Autodesk Inventor part; units mm, degrees
(part 3 of 4)
  arc A252 (17.6649, -16.827) -> (17.6214, -17.1875) centre (17.8848, -17.0365) ccw projected
  arc A253 (18.3289, -18.7127) -> (17.6214, -17.1875) centre (9.134, -22.0513) ccw projected
  arc A254 (17.8536, -19.1667) -> (18.3289, -18.7127) centre (0, 0) ccw projected
  arc A255 (16.3624, -18.39) -> (17.8536, -19.1667) centre (21.6099, -10.1343) ccw projected
  arc A256 (16.3624, -18.39) -> (16.0003, -18.4171) centre (16.1995, -18.6463) ccw projected
  arc A257 (15.9306, -18.4775) -> (16.0003, -18.4171) centre (0, 0) ccw projected
  arc A258 (15.9306, -18.4775) -> (15.8518, -18.8319) centre (16.1289, -18.7075) ccw projected
  arc A259 (16.4065, -20.4191) -> (15.8518, -18.8319) centre (6.9286, -22.8404) ccw projected
  arc A260 (15.889, -20.8243) -> (16.4065, -20.4191) centre (0, 0) ccw projected
  arc A261 (14.4811, -19.9053) -> (15.889, -20.8243) centre (20.5125, -12.2036) ccw projected
  arc A262 (14.4811, -19.9053) -> (14.1181, -19.8967) centre (14.2938, -20.1444) ccw projected
  arc A263 (14.0427, -19.95) -> (14.1181, -19.8967) centre (0, 0) ccw projected
  arc A264 (14.0427, -19.95) -> (13.9297, -20.295) centre (14.2175, -20.1983) ccw projected
  arc A265 (14.326, -21.9289) -> (13.9297, -20.295) centre (4.6565, -23.4096) ccw projected
  arc A266 (13.7713, -22.2814) -> (14.326, -21.9289) centre (0, 0) ccw projected
  arc A267 (12.4603, -21.2288) -> (13.7713, -22.2814) centre (19.2175, -14.1555) ccw projected
  arc A268 (12.4603, -21.2288) -> (12.0999, -21.1847) centre (12.2505, -21.4484) ccw projected
  arc A269 (12.0197, -21.2303) -> (12.0999, -21.1847) centre (0, 0) ccw projected
  arc A270 (12.0197, -21.2303) -> (11.8733, -21.5626) centre (12.1693, -21.4946) ccw projected
  arc A271 (12.1076, -23.2275) -> (11.8733, -21.5626) centre (2.3395, -23.7533) ccw projected
  arc A272 (11.5211, -23.524) -> (12.1076, -23.2275) centre (0, 0) ccw projected
  arc A273 (10.3195, -22.3479) -> (11.5211, -23.524) centre (17.7375, -15.9709) ccw projected
  arc A274 (10.3195, -22.3479) -> (9.9652, -22.2687) centre (10.0892, -22.5459) ccw projected
  arc A275 (9.8809, -22.3062) -> (9.9652, -22.2687) centre (0, 0) ccw projected
  arc A276 (9.8809, -22.3062) -> (9.7026, -22.6226) centre (10.0039, -22.5839) ccw projected
  arc A277 (9.7726, -24.3024) -> (9.7026, -22.6226) centre (0, -23.8682) ccw projected
  arc A278 (9.1598, -24.54) -> (9.7726, -24.3024) centre (0, 0) ccw projected
  arc A279 (8.0793, -23.2518) -> (9.1598, -24.54) centre (16.0867, -17.6326) ccw projected
  arc A280 (8.0793, -23.2518) -> (7.7345, -23.1382) centre (7.8307, -23.4262) ccw projected
  arc A281 (7.6469, -23.1673) -> (7.7345, -23.1382) centre (0, 0) ccw projected
  arc A282 (7.6469, -23.1673) -> (7.4385, -23.4646) centre (7.7421, -23.4557) ccw projected
  arc A283 (7.3435, -25.1433) -> (7.4385, -23.4646) centre (-2.3395, -23.7533) ccw projected
  arc A284 (6.7104, -25.3196) -> (7.3435, -25.1433) centre (0, 0) ccw projected
  arc A285 (5.7614, -23.9317) -> (6.7104, -25.3196) centre (14.2809, -19.1245) ccw projected
  arc A286 (5.7614, -23.9317) -> (5.4293, -23.7849) centre (5.4969, -24.081) ccw projected
  arc A287 (5.3393, -23.8053) -> (5.4293, -23.7849) centre (0, 0) ccw projected
  arc A288 (5.3393, -23.8053) -> (5.1028, -24.0808) centre (5.4057, -24.1016) ccw projected
  arc A289 (4.8437, -25.742) -> (5.1028, -24.0808) centre (-4.6565, -23.4096) ccw projected
  arc A290 (4.1963, -25.8554) -> (4.8437, -25.742) centre (0, 0) ccw projected
  arc A291 (3.3879, -24.3812) -> (4.1963, -25.8554) centre (12.3376, -20.4322) ccw projected
  arc A292 (3.3879, -24.3812) -> (3.0718, -24.2025) centre (3.11, -24.5038) ccw projected
  arc A293 (2.9802, -24.214) -> (3.0718, -24.2025) centre (0, 0) ccw projected
  arc A294 (2.9802, -24.214) -> (2.7179, -24.465) centre (3.0173, -24.5154) ccw projected
  arc A295 (2.2972, -26.0928) -> (2.7179, -24.465) centre (-6.9286, -22.8404) ccw projected
  arc A296 (1.6418, -26.1422) -> (2.2972, -26.0928) centre (0, 0) ccw projected
  arc A297 (0.9818, -24.5959) -> (1.6418, -26.1422) centre (10.2755, -21.5431) ccw projected
  arc A298 (0.9818, -24.5959) -> (0.6848, -24.3871) centre (0.6933, -24.6907) ccw projected
  arc A299 (0.5925, -24.3895) -> (0.6848, -24.3871) centre (0, 0) ccw projected
  arc A300 (0.5925, -24.3895) -> (0.3068, -24.6136) centre (0.5999, -24.6931) ccw projected
  arc A301 (-0.2714, -26.1923) -> (0.3068, -24.6136) centre (-9.134, -22.0513) ccw projected
  arc A302 (-0.9285, -26.1773) -> (-0.2714, -26.1923) centre (0, 0) ccw projected
  arc A303 (-1.4337, -24.5737) -> (-0.9285, -26.1773) centre (8.1145, -22.4465) ccw projected
  arc A304 (-1.4337, -24.5737) -> (-1.7089, -24.3368) centre (-1.7302, -24.6397) ccw projected
  arc A305 (-1.8009, -24.3301) -> (-1.7089, -24.3368) centre (0, 0) ccw projected
  arc A306 (-1.8009, -24.3301) -> (-2.1072, -24.5251) centre (-1.8234, -24.633) ccw projected
  arc A307 (-2.8374, -26.0396) -> (-2.1072, -24.5251) centre (-11.2514, -21.0499) ccw projected
  arc A308 (-3.4898, -25.9602) -> (-2.8374, -26.0396) centre (0, 0) ccw projected
  arc A309 (-3.8355, -24.3148) -> (-3.4898, -25.9602) centre (5.8752, -23.1338) ccw projected
  arc A310 (-3.8355, -24.3148) -> (-4.0861, -24.0521) centre (-4.137, -24.3515) ccw projected
  arc A311 (-4.177, -24.0365) -> (-4.0861, -24.0521) centre (0, 0) ccw projected
  arc A312 (-4.177, -24.0365) -> (-4.501, -24.2005) centre (-4.229, -24.3357) ccw projected
  arc A313 (-5.3761, -25.6361) -> (-4.501, -24.2005) centre (-13.2605, -19.8457) ccw projected
  arc A314 (-6.0176, -25.4932) -> (-5.3761, -25.6361) centre (0, 0) ccw projected
  arc A315 (-6.2003, -23.8218) -> (-6.0176, -25.4932) centre (3.5794, -23.5983) ccw projected
  arc A316 (-6.2003, -23.8218) -> (-6.4239, -23.5358) centre (-6.5039, -23.8287) ccw projected
  arc A317 (-6.5129, -23.5113) -> (-6.4239, -23.5358) centre (0, 0) ccw projected
  arc A318 (-6.5129, -23.5113) -> (-6.8514, -23.6428) centre (-6.594, -23.804) ccw projected
  arc A319 (-7.863, -24.9857) -> (-6.8514, -23.6428) centre (-15.1418, -18.4504) ccw projected
  arc A320 (-8.4873, -24.7806) -> (-7.863, -24.9857) centre (0, 0) ccw projected
  arc A321 (-8.5054, -23.0994) -> (-8.4873, -24.7806) centre (1.2492, -23.8355) ccw projected
  arc A322 (-8.5054, -23.0994) -> (-8.6999, -22.7928) centre (-8.8082, -23.0765) ccw projected
  arc A323 (-8.7861, -22.7597) -> (-8.6999, -22.7928) centre (0, 0) ccw projected
  arc A324 (-8.7861, -22.7597) -> (-9.1358, -22.8574) centre (-8.8954, -23.043) ccw projected
  arc A325 (-10.2741, -24.0947) -> (-9.1358, -22.8574) centre (-16.8774, -16.8774) ccw projected
  arc A326 (-10.8754, -23.8294) -> (-10.2741, -24.0947) centre (0, 0) ccw projected
  arc A327 (-10.7286, -22.1544) -> (-10.8754, -23.8294) centre (-1.0931, -23.8431) ccw projected
  arc A328 (-10.7286, -22.1544) -> (-10.8921, -21.8303) centre (-11.0277, -22.102) ccw projected
  arc A329 (-10.9746, -21.7889) -> (-10.8921, -21.8303) centre (0, 0) ccw projected
  arc A330 (-10.9746, -21.7889) -> (-11.3322, -21.8518) centre (-11.1112, -22.0602) ccw projected
  arc A331 (-12.5863, -22.9716) -> (-11.3322, -21.8518) centre (-18.4504, -15.1418) ccw projected
  arc A332 (-13.1587, -22.6486) -> (-12.5863, -22.9716) centre (0, 0) ccw projected
  arc A333 (-12.8484, -20.9962) -> (-13.1587, -22.6486) centre (-3.4249, -23.6212) ccw projected
  arc A334 (-12.8484, -20.9962) -> (-12.9794, -20.6576) centre (-13.141, -20.9147) ccw projected
  arc A335 (-13.0574, -20.6083) -> (-12.9794, -20.6576) centre (0, 0) ccw projected
  arc A336 (-13.0574, -20.6083) -> (-13.4195, -20.6359) centre (-13.22, -20.8648) ccw projected
  arc A337 (-14.7773, -21.6274) -> (-13.4195, -20.6359) centre (-19.8457, -13.2605) ccw projected
  arc A338 (-15.3153, -21.2498) -> (-14.7773, -21.6274) centre (0, 0) ccw projected
  arc A339 (-14.8445, -19.6357) -> (-15.3153, -21.2498) centre (-5.7237, -23.1717) ccw projected
  arc A340 (-14.8445, -19.6357) -> (-14.9417, -19.2859) centre (-15.1277, -19.5259) ccw projected
  arc A341 (-15.0145, -19.2292) -> (-14.9417, -19.2859) centre (0, 0) ccw projected
  arc A342 (-15.0145, -19.2292) -> (-15.3775, -19.2212) centre (-15.2014, -19.4686) ccw projected
  arc A343 (-16.826, -20.0748) -> (-15.3775, -19.2212) centre (-21.0499, -11.2514) ccw projected
  arc A344 (-17.3244, -19.6463) -> (-16.826, -20.0748) centre (0, 0) ccw projected
  arc A345 (-16.6977, -18.0862) -> (-17.3244, -19.6463) centre (-7.9674, -22.4991) ccw projected
  arc A346 (-16.6977, -18.0862) -> (-16.7601, -17.7285) centre (-16.9687, -17.9492) ccw projected
  arc A347 (-16.827, -17.6649) -> (-16.7601, -17.7285) centre (0, 0) ccw projected
  arc A348 (-16.827, -17.6649) -> (-17.1875, -17.6214) centre (-17.0365, -17.8848) ccw projected
  arc A349 (-18.7127, -18.3289) -> (-17.1875, -17.6214) centre (-22.0513, -9.134) ccw projected
  arc A350 (-19.1667, -17.8536) -> (-18.7127, -18.3289) centre (0, 0) ccw projected
  arc A351 (-18.39, -16.3624) -> (-19.1667, -17.8536) centre (-10.1343, -21.6099) ccw projected
  arc A352 (-18.39, -16.3624) -> (-18.4171, -16.0003) centre (-18.6463, -16.1995) ccw projected
  arc A353 (-18.4775, -15.9306) -> (-18.4171, -16.0003) centre (0, 0) ccw projected
  arc A354 (-18.4775, -15.9306) -> (-18.8319, -15.8518) centre (-18.7075, -16.1289) ccw projected
  arc A355 (-20.4191, -16.4065) -> (-18.8319, -15.8518) centre (-22.8404, -6.9286) ccw projected
  arc A356 (-20.8243, -15.889) -> (-20.4191, -16.4065) centre (0, 0) ccw projected
  arc A357 (-19.9053, -14.4811) -> (-20.8243, -15.889) centre (-12.2036, -20.5125) ccw projected
  arc A358 (-19.9053, -14.4811) -> (-19.8967, -14.1181) centre (-20.1444, -14.2938) ccw projected
  arc A359 (-19.95, -14.0427) -> (-19.8967, -14.1181) centre (0, 0) ccw projected
  arc A360 (-19.95, -14.0427) -> (-20.295, -13.9297) centre (-20.1983, -14.2175) ccw projected
  arc A361 (-21.9289, -14.326) -> (-20.295, -13.9297) centre (-23.4096, -4.6565) ccw projected
  arc A362 (-22.2814, -13.7713) -> (-21.9289, -14.326) centre (0, 0) ccw projected
  arc A363 (-21.2288, -12.4603) -> (-22.2814, -13.7713) centre (-14.1555, -19.2175) ccw projected
  arc A364 (-21.2288, -12.4603) -> (-21.1847, -12.0999) centre (-21.4484, -12.2505) ccw projected
  arc A365 (-21.2303, -12.0197) -> (-21.1847, -12.0999) centre (0, 0) ccw projected
  arc A366 (-21.2303, -12.0197) -> (-21.5626, -11.8733) centre (-21.4946, -12.1693) ccw projected
  arc A367 (-23.2275, -12.1076) -> (-21.5626, -11.8733) centre (-23.7533, -2.3395) ccw projected
  arc A368 (-23.524, -11.5211) -> (-23.2275, -12.1076) centre (0, 0) ccw projected
  arc A369 (-22.3479, -10.3195) -> (-23.524, -11.5211) centre (-15.9709, -17.7375) ccw projected
  arc A370 (-22.3479, -10.3195) -> (-22.2687, -9.9652) centre (-22.5459, -10.0892) ccw projected
  arc A371 (-22.3062, -9.8809) -> (-22.2687, -9.9652) centre (0, 0) ccw projected
  arc A372 (-22.3062, -9.8809) -> (-22.6226, -9.7026) centre (-22.5839, -10.0039) ccw projected
  arc A373 (-24.3024, -9.7726) -> (-22.6226, -9.7026) centre (-23.8682, 0) ccw projected
  arc A374 (-24.54, -9.1598) -> (-24.3024, -9.7726) centre (0, 0) ccw projected
  arc A375 (-23.2518, -8.0793) -> (-24.54, -9.1598) centre (-17.6326, -16.0867) ccw projected
  arc A376 (-23.2518, -8.0793) -> (-23.1382, -7.7345) centre (-23.4262, -7.8307) ccw projected
  arc A377 (-23.1673, -7.6469) -> (-23.1382, -7.7345) centre (0, 0) ccw projected
  arc A378 (-23.1673, -7.6469) -> (-23.4646, -7.4385) centre (-23.4557, -7.7421) ccw projected
  arc A379 (-25.1433, -7.3435) -> (-23.4646, -7.4385) centre (-23.7533, 2.3395) ccw projected
  arc A380 (-25.3196, -6.7104) -> (-25.1433, -7.3435) centre (0, 0) ccw projected
  arc A381 (-23.9317, -5.7614) -> (-25.3196, -6.7104) centre (-19.1245, -14.2809) ccw projected
  arc A382 (-23.9317, -5.7614) -> (-23.7849, -5.4293) centre (-24.081, -5.4969) ccw projected
  arc A383 (-23.8053, -5.3393) -> (-23.7849, -5.4293) centre (0, 0) ccw projected
  arc A384 (-23.8053, -5.3393) -> (-24.0808, -5.1028) centre (-24.1016, -5.4057) ccw projected
  point P0 (0, 0)
extrude "Extrusion5" add sketch "Sketch5" along normal blind 1.27
sketch "Sketch6" plane through (0, 0, 25.781) normal (0, 0, -1) x (-1, 0, 0)
  circle A0 centre (0, 0) radius 29.475
  constraints: 1 centre point, 1 coincident
extrude "Extrusion6" add sketch "Sketch6" along normal blind 1.27
sketch "Sketch7" plane through (0, 0, 32.131) normal (0, 0, 1) x (1, 0, 0)
  arc A0 (24.0808, -5.1028) -> (23.8053, -5.3393) centre (24.1016, -5.4057) ccw projected
  arc A1 (23.7849, -5.4293) -> (23.8053, -5.3393) centre (0, 0) ccw projected
  arc A2 (23.7849, -5.4293) -> (23.9317, -5.7614) centre (24.081, -5.4969) ccw projected
  arc A3 (25.3196, -6.7104) -> (23.9317, -5.7614) centre (19.1245, -14.2809) ccw projected
  arc A4 (25.1433, -7.3435) -> (25.3196, -6.7104) centre (0, 0) ccw projected
  arc A5 (23.4646, -7.4385) -> (25.1433, -7.3435) centre (23.7533, 2.3395) ccw projected
  arc A6 (23.4646, -7.4385) -> (23.1673, -7.6469) centre (23.4557, -7.7421) ccw projected
  arc A7 (23.1382, -7.7345) -> (23.1673, -7.6469) centre (0, 0) ccw projected
  arc A8 (23.1382, -7.7345) -> (23.2518, -8.0793) centre (23.4262, -7.8307) ccw projected
  arc A9 (24.54, -9.1598) -> (23.2518, -8.0793) centre (17.6326, -16.0867) ccw projected
  arc A10 (24.3024, -9.7726) -> (24.54, -9.1598) centre (0, 0) ccw projected
  arc A11 (22.6226, -9.7026) -> (24.3024, -9.7726) centre (23.8682, 0) ccw projected
  arc A12 (22.6226, -9.7026) -> (22.3062, -9.8809) centre (22.5839, -10.0039) ccw projected
  arc A13 (22.2687, -9.9652) -> (22.3062, -9.8809) centre (0, 0) ccw projected
  arc A14 (22.2687, -9.9652) -> (22.3479, -10.3195) centre (22.5459, -10.0892) ccw projected
  arc A15 (23.524, -11.5211) -> (22.3479, -10.3195) centre (15.9709, -17.7375) ccw projected
  arc A16 (23.2275, -12.1076) -> (23.524, -11.5211) centre (0, 0) ccw projected
  arc A17 (21.5626, -11.8733) -> (23.2275, -12.1076) centre (23.7533, -2.3395) ccw projected
  arc A18 (21.5626, -11.8733) -> (21.2303, -12.0197) centre (21.4946, -12.1693) ccw projected
  arc A19 (21.1847, -12.0999) -> (21.2303, -12.0197) centre (0, 0) ccw projected
  arc A20 (21.1847, -12.0999) -> (21.2288, -12.4603) centre (21.4484, -12.2505) ccw projected
  arc A21 (22.2814, -13.7713) -> (21.2288, -12.4603) centre (14.1555, -19.2175) ccw projected
  arc A22 (21.9289, -14.326) -> (22.2814, -13.7713) centre (0, 0) ccw projected
  arc A23 (20.295, -13.9297) -> (21.9289, -14.326) centre (23.4096, -4.6565) ccw projected
  arc A24 (20.295, -13.9297) -> (19.95, -14.0427) centre (20.1983, -14.2175) ccw projected
  arc A25 (19.8967, -14.1181) -> (19.95, -14.0427) centre (0, 0) ccw projected
  arc A26 (19.8967, -14.1181) -> (19.9053, -14.4811) centre (20.1444, -14.2938) ccw projected
  arc A27 (20.8243, -15.889) -> (19.9053, -14.4811) centre (12.2036, -20.5125) ccw projected
  arc A28 (20.4191, -16.4065) -> (20.8243, -15.889) centre (0, 0) ccw projected
  arc A29 (18.8319, -15.8518) -> (20.4191, -16.4065) centre (22.8404, -6.9286) ccw projected
  arc A30 (18.8319, -15.8518) -> (18.4775, -15.9306) centre (18.7075, -16.1289) ccw projected
  arc A31 (18.4171, -16.0003) -> (18.4775, -15.9306) centre (0, 0) ccw projected
  arc A32 (18.4171, -16.0003) -> (18.39, -16.3624) centre (18.6463, -16.1995) ccw projected
  arc A33 (19.1667, -17.8536) -> (18.39, -16.3624) centre (10.1343, -21.6099) ccw projected
  arc A34 (18.7127, -18.3289) -> (19.1667, -17.8536) centre (0, 0) ccw projected
  arc A35 (17.1875, -17.6214) -> (18.7127, -18.3289) centre (22.0513, -9.134) ccw projected
  arc A36 (17.1875, -17.6214) -> (16.827, -17.6649) centre (17.0365, -17.8848) ccw projected
  arc A37 (16.7601, -17.7285) -> (16.827, -17.6649) centre (0, 0) ccw projected
  arc A38 (16.7601, -17.7285) -> (16.6977, -18.0862) centre (16.9687, -17.9492) ccw projected
  arc A39 (17.3244, -19.6463) -> (16.6977, -18.0862) centre (7.9674, -22.4991) ccw projected
  arc A40 (16.826, -20.0748) -> (17.3244, -19.6463) centre (0, 0) ccw projected
  arc A41 (15.3775, -19.2212) -> (16.826, -20.0748) centre (21.0499, -11.2514) ccw projected
  arc A42 (15.3775, -19.2212) -> (15.0145, -19.2292) centre (15.2014, -19.4686) ccw projected
  arc A43 (14.9417, -19.2859) -> (15.0145, -19.2292) centre (0, 0) ccw projected
  arc A44 (14.9417, -19.2859) -> (14.8445, -19.6357) centre (15.1277, -19.5259) ccw projected
  arc A45 (15.3153, -21.2498) -> (14.8445, -19.6357) centre (5.7237, -23.1717) ccw projected
  arc A46 (14.7773, -21.6274) -> (15.3153, -21.2498) centre (0, 0) ccw projected
  arc A47 (13.4195, -20.6359) -> (14.7773, -21.6274) centre (19.8457, -13.2605) ccw projected
  arc A48 (13.4195, -20.6359) -> (13.0574, -20.6083) centre (13.22, -20.8648) ccw projected
  arc A49 (12.9794, -20.6576) -> (13.0574, -20.6083) centre (0, 0) ccw projected
  arc A50 (12.9794, -20.6576) -> (12.8484, -20.9962) centre (13.141, -20.9147) ccw projected
  arc A51 (13.1587, -22.6486) -> (12.8484, -20.9962) centre (3.4249, -23.6212) ccw projected
  arc A52 (12.5863, -22.9716) -> (13.1587, -22.6486) centre (0, 0) ccw projected
  arc A53 (11.3322, -21.8518) -> (12.5863, -22.9716) centre (18.4504, -15.1418) ccw projected
  arc A54 (11.3322, -21.8518) -> (10.9746, -21.7889) centre (11.1112, -22.0602) ccw projected
  arc A55 (10.8921, -21.8303) -> (10.9746, -21.7889) centre (0, 0) ccw projected
  arc A56 (10.8921, -21.8303) -> (10.7286, -22.1544) centre (11.0277, -22.102) ccw projected
  arc A57 (10.8754, -23.8294) -> (10.7286, -22.1544) centre (1.0931, -23.8431) ccw projected
  arc A58 (10.2741, -24.0947) -> (10.8754, -23.8294) centre (0, 0) ccw projected
  arc A59 (9.1358, -22.8574) -> (10.2741, -24.0947) centre (16.8774, -16.8774) ccw projected
  arc A60 (9.1358, -22.8574) -> (8.7861, -22.7597) centre (8.8954, -23.043) ccw projected
  arc A61 (8.6999, -22.7928) -> (8.7861, -22.7597) centre (0, 0) ccw projected
  arc A62 (8.6999, -22.7928) -> (8.5054, -23.0994) centre (8.8082, -23.0765) ccw projected
  arc A63 (8.4873, -24.7806) -> (8.5054, -23.0994) centre (-1.2492, -23.8355) ccw projected
  arc A64 (7.863, -24.9857) -> (8.4873, -24.7806) centre (0, 0) ccw projected
  arc A65 (6.8514, -23.6428) -> (7.863, -24.9857) centre (15.1418, -18.4504) ccw projected
  arc A66 (6.8514, -23.6428) -> (6.5129, -23.5113) centre (6.594, -23.804) ccw projected
  arc A67 (6.4239, -23.5358) -> (6.5129, -23.5113) centre (0, 0) ccw projected
  arc A68 (6.4239, -23.5358) -> (6.2003, -23.8218) centre (6.5039, -23.8287) ccw projected
  arc A69 (6.0176, -25.4932) -> (6.2003, -23.8218) centre (-3.5794, -23.5983) ccw projected
  arc A70 (5.3761, -25.6361) -> (6.0176, -25.4932) centre (0, 0) ccw projected
  arc A71 (4.501, -24.2005) -> (5.3761, -25.6361) centre (13.2605, -19.8457) ccw projected
  arc A72 (4.501, -24.2005) -> (4.177, -24.0365) centre (4.229, -24.3357) ccw projected
  arc A73 (4.0861, -24.0521) -> (4.177, -24.0365) centre (0, 0) ccw projected
  arc A74 (4.0861, -24.0521) -> (3.8355, -24.3148) centre (4.137, -24.3515) ccw projected
  arc A75 (3.4898, -25.9602) -> (3.8355, -24.3148) centre (-5.8752, -23.1338) ccw projected
  arc A76 (2.8374, -26.0396) -> (3.4898, -25.9602) centre (0, 0) ccw projected
  arc A77 (2.1072, -24.5251) -> (2.8374, -26.0396) centre (11.2514, -21.0499) ccw projected
  arc A78 (2.1072, -24.5251) -> (1.8009, -24.3301) centre (1.8234, -24.633) ccw projected
  arc A79 (1.7089, -24.3368) -> (1.8009, -24.3301) centre (0, 0) ccw projected
  arc A80 (1.7089, -24.3368) -> (1.4337, -24.5737) centre (1.7302, -24.6397) ccw projected
  arc A81 (0.9285, -26.1773) -> (1.4337, -24.5737) centre (-8.1145, -22.4465) ccw projected
  arc A82 (0.2714, -26.1923) -> (0.9285, -26.1773) centre (0, 0) ccw projected
  arc A83 (-0.3068, -24.6136) -> (0.2714, -26.1923) centre (9.134, -22.0513) ccw projected
  arc A84 (-0.3068, -24.6136) -> (-0.5925, -24.3895) centre (-0.5999, -24.6931) ccw projected
  arc A85 (-0.6848, -24.3871) -> (-0.5925, -24.3895) centre (0, 0) ccw projected
  arc A86 (-0.6848, -24.3871) -> (-0.9818, -24.5959) centre (-0.6933, -24.6907) ccw projected
  arc A87 (-1.6418, -26.1422) -> (-0.9818, -24.5959) centre (-10.2755, -21.5431) ccw projected
  arc A88 (-2.2972, -26.0928) -> (-1.6418, -26.1422) centre (0, 0) ccw projected
  arc A89 (-2.7179, -24.465) -> (-2.2972, -26.0928) centre (6.9286, -22.8404) ccw projected
  arc A90 (-2.7179, -24.465) -> (-2.9802, -24.214) centre (-3.0173, -24.5154) ccw projected
  arc A91 (-3.0718, -24.2025) -> (-2.9802, -24.214) centre (0, 0) ccw projected
  arc A92 (-3.0718, -24.2025) -> (-3.3879, -24.3812) centre (-3.11, -24.5038) ccw projected
  arc A93 (-4.1963, -25.8554) -> (-3.3879, -24.3812) centre (-12.3376, -20.4322) ccw projected
  arc A94 (-4.8437, -25.742) -> (-4.1963, -25.8554) centre (0, 0) ccw projected
  arc A95 (-5.1028, -24.0808) -> (-4.8437, -25.742) centre (4.6565, -23.4096) ccw projected
  arc A96 (-5.1028, -24.0808) -> (-5.3393, -23.8053) centre (-5.4057, -24.1016) ccw projected
  arc A97 (-5.4293, -23.7849) -> (-5.3393, -23.8053) centre (0, 0) ccw projected
  arc A98 (-5.4293, -23.7849) -> (-5.7614, -23.9317) centre (-5.4969, -24.081) ccw projected
  arc A99 (-6.7104, -25.3196) -> (-5.7614, -23.9317) centre (-14.2809, -19.1245) ccw projected
  arc A100 (-7.3435, -25.1433) -> (-6.7104, -25.3196) centre (0, 0) ccw projected
  arc A101 (-7.4385, -23.4646) -> (-7.3435, -25.1433) centre (2.3395, -23.7533) ccw projected
  arc A102 (-7.4385, -23.4646) -> (-7.6469, -23.1673) centre (-7.7421, -23.4557) ccw projected
  arc A103 (-7.7345, -23.1382) -> (-7.6469, -23.1673) centre (0, 0) ccw projected
  arc A104 (-7.7345, -23.1382) -> (-8.0793, -23.2518) centre (-7.8307, -23.4262) ccw projected
  arc A105 (-9.1598, -24.54) -> (-8.0793, -23.2518) centre (-16.0867, -17.6326) ccw projected
  arc A106 (-9.7726, -24.3024) -> (-9.1598, -24.54) centre (0, 0) ccw projected
  arc A107 (-9.7026, -22.6226) -> (-9.7726, -24.3024) centre (0, -23.8682) ccw projected
  arc A108 (-9.7026, -22.6226) -> (-9.8809, -22.3062) centre (-10.0039, -22.5839) ccw projected
  arc A109 (-9.9652, -22.2687) -> (-9.8809, -22.3062) centre (0, 0) ccw projected
  arc A110 (-9.9652, -22.2687) -> (-10.3195, -22.3479) centre (-10.0892, -22.5459) ccw projected
  arc A111 (-11.5211, -23.524) -> (-10.3195, -22.3479) centre (-17.7375, -15.9709) ccw projected
  arc A112 (-12.1076, -23.2275) -> (-11.5211, -23.524) centre (0, 0) ccw projected
  arc A113 (-11.8733, -21.5626) -> (-12.1076, -23.2275) centre (-2.3395, -23.7533) ccw projected
  arc A114 (-11.8733, -21.5626) -> (-12.0197, -21.2303) centre (-12.1693, -21.4946) ccw projected
  arc A115 (-12.0999, -21.1847) -> (-12.0197, -21.2303) centre (0, 0) ccw projected
  arc A116 (-12.0999, -21.1847) -> (-12.4603, -21.2288) centre (-12.2505, -21.4484) ccw projected
  arc A117 (-13.7713, -22.2814) -> (-12.4603, -21.2288) centre (-19.2175, -14.1555) ccw projected
  arc A118 (-14.326, -21.9289) -> (-13.7713, -22.2814) centre (0, 0) ccw projected
  arc A119 (-13.9297, -20.295) -> (-14.326, -21.9289) centre (-4.6565, -23.4096) ccw projected
  arc A120 (-13.9297, -20.295) -> (-14.0427, -19.95) centre (-14.2175, -20.1983) ccw projected
  arc A121 (-14.1181, -19.8967) -> (-14.0427, -19.95) centre (0, 0) ccw projected
  arc A122 (-14.1181, -19.8967) -> (-14.4811, -19.9053) centre (-14.2938, -20.1444) ccw projected
  arc A123 (-15.889, -20.8243) -> (-14.4811, -19.9053) centre (-20.5125, -12.2036) ccw projected
  arc A124 (-16.4065, -20.4191) -> (-15.889, -20.8243) centre (0, 0) ccw projected
  arc A125 (-15.8518, -18.8319) -> (-16.4065, -20.4191) centre (-6.9286, -22.8404) ccw projected
  arc A126 (-15.8518, -18.8319) -> (-15.9306, -18.4775) centre (-16.1289, -18.7075) ccw projected
  arc A127 (-16.0003, -18.4171) -> (-15.9306, -18.4775) centre (0, 0) ccw projected
  arc A128 (-16.0003, -18.4171) -> (-16.3624, -18.39) centre (-16.1995, -18.6463) ccw projected
  arc A129 (-17.8536, -19.1667) -> (-16.3624, -18.39) centre (-21.6099, -10.1343) ccw projected
  arc A130 (-18.3289, -18.7127) -> (-17.8536, -19.1667) centre (0, 0) ccw projected
  arc A131 (-17.6214, -17.1875) -> (-18.3289, -18.7127) centre (-9.134, -22.0513) ccw projected
  arc A132 (-17.6214, -17.1875) -> (-17.6649, -16.827) centre (-17.8848, -17.0365) ccw projected
  arc A133 (-17.7285, -16.7601) -> (-17.6649, -16.827) centre (0, 0) ccw projected
  arc A134 (-17.7285, -16.7601) -> (-18.0862, -16.6977) centre (-17.9492, -16.9687) ccw projected
  arc A135 (-19.6463, -17.3244) -> (-18.0862, -16.6977) centre (-22.4991, -7.9674) ccw projected
  arc A136 (-20.0748, -16.826) -> (-19.6463, -17.3244) centre (0, 0) ccw projected
  arc A137 (-19.2212, -15.3775) -> (-20.0748, -16.826) centre (-11.2514, -21.0499) ccw projected
  arc A138 (-19.2212, -15.3775) -> (-19.2292, -15.0145) centre (-19.4686, -15.2014) ccw projected
  arc A139 (-19.2859, -14.9417) -> (-19.2292, -15.0145) centre (0, 0) ccw projected
  arc A140 (-19.2859, -14.9417) -> (-19.6357, -14.8445) centre (-19.5259, -15.1277) ccw projected
  arc A141 (-21.2498, -15.3153) -> (-19.6357, -14.8445) centre (-23.1717, -5.7237) ccw projected
  arc A142 (-21.6274, -14.7773) -> (-21.2498, -15.3153) centre (0, 0) ccw projected
  arc A143 (-20.6359, -13.4195) -> (-21.6274, -14.7773) centre (-13.2605, -19.8457) ccw projected
  arc A144 (-20.6359, -13.4195) -> (-20.6083, -13.0574) centre (-20.8648, -13.22) ccw projected
  arc A145 (-20.6576, -12.9794) -> (-20.6083, -13.0574) centre (0, 0) ccw projected
  arc A146 (-20.6576, -12.9794) -> (-20.9962, -12.8484) centre (-20.9147, -13.141) ccw projected
  arc A147 (-22.6486, -13.1587) -> (-20.9962, -12.8484) centre (-23.6212, -3.4249) ccw projected
  arc A148 (-22.9716, -12.5863) -> (-22.6486, -13.1587) centre (0, 0) ccw projected
  arc A149 (-21.8518, -11.3322) -> (-22.9716, -12.5863) centre (-15.1418, -18.4504) ccw projected
  arc A150 (-21.8518, -11.3322) -> (-21.7889, -10.9746) centre (-22.0602, -11.1112) ccw projected
  arc A151 (-21.8303, -10.8921) -> (-21.7889, -10.9746) centre (0, 0) ccw projected
  arc A152 (-21.8303, -10.8921) -> (-22.1544, -10.7286) centre (-22.102, -11.0277) ccw projected
  arc A153 (-23.8294, -10.8754) -> (-22.1544, -10.7286) centre (-23.8431, -1.0931) ccw projected
  arc A154 (-24.0947, -10.2741) -> (-23.8294, -10.8754) centre (0, 0) ccw projected
  arc A155 (-22.8574, -9.1358) -> (-24.0947, -10.2741) centre (-16.8774, -16.8774) ccw projected
  arc A156 (-22.8574, -9.1358) -> (-22.7597, -8.7861) centre (-23.043, -8.8954) ccw projected
  arc A157 (-22.7928, -8.6999) -> (-22.7597, -8.7861) centre (0, 0) ccw projected
  arc A158 (-22.7928, -8.6999) -> (-23.0994, -8.5054) centre (-23.0765, -8.8082) ccw projected
  arc A159 (-24.7806, -8.4873) -> (-23.0994, -8.5054) centre (-23.8355, 1.2492) ccw projected
  arc A160 (-24.9857, -7.863) -> (-24.7806, -8.4873) centre (0, 0) ccw projected
  arc A161 (-23.6428, -6.8514) -> (-24.9857, -7.863) centre (-18.4504, -15.1418) ccw projected
  arc A162 (-23.6428, -6.8514) -> (-23.5113, -6.5129) centre (-23.804, -6.594) ccw projected
  arc A163 (-23.5358, -6.4239) -> (-23.5113, -6.5129) centre (0, 0) ccw projected
  arc A164 (-23.5358, -6.4239) -> (-23.8218, -6.2003) centre (-23.8287, -6.5039) ccw projected
  arc A165 (-25.4932, -6.0176) -> (-23.8218, -6.2003) centre (-23.5983, 3.5794) ccw projected
  arc A166 (-25.6361, -5.3761) -> (-25.4932, -6.0176) centre (0, 0) ccw projected
  arc A167 (-24.2005, -4.501) -> (-25.6361, -5.3761) centre (-19.8457, -13.2605) ccw projected
  arc A168 (-24.2005, -4.501) -> (-24.0365, -4.177) centre (-24.3357, -4.229) ccw projected
  arc A169 (-24.0521, -4.0861) -> (-24.0365, -4.177) centre (0, 0) ccw projected
  arc A170 (-24.0521, -4.0861) -> (-24.3148, -3.8355) centre (-24.3515, -4.137) ccw projected
  arc A171 (-25.9602, -3.4898) -> (-24.3148, -3.8355) centre (-23.1338, 5.8752) ccw projected
  arc A172 (-26.0396, -2.8374) -> (-25.9602, -3.4898) centre (0, 0) ccw projected
  arc A173 (-24.5251, -2.1072) -> (-26.0396, -2.8374) centre (-21.0499, -11.2514) ccw projected
  arc A174 (-24.5251, -2.1072) -> (-24.3301, -1.8009) centre (-24.633, -1.8234) ccw projected
  arc A175 (-24.3368, -1.7089) -> (-24.3301, -1.8009) centre (0, 0) ccw projected
  arc A176 (-24.3368, -1.7089) -> (-24.5737, -1.4337) centre (-24.6397, -1.7302) ccw projected
  arc A177 (-26.1773, -0.9285) -> (-24.5737, -1.4337) centre (-22.4465, 8.1145) ccw projected
  arc A178 (-26.1923, -0.2714) -> (-26.1773, -0.9285) centre (0, 0) ccw projected
  arc A179 (-24.6136, 0.3068) -> (-26.1923, -0.2714) centre (-22.0513, -9.134) ccw projected
  arc A180 (-24.6136, 0.3068) -> (-24.3895, 0.5925) centre (-24.6931, 0.5999) ccw projected
  arc A181 (-24.3871, 0.6848) -> (-24.3895, 0.5925) centre (0, 0) ccw projected
  arc A182 (-24.3871, 0.6848) -> (-24.5959, 0.9818) centre (-24.6907, 0.6933) ccw projected
  arc A183 (-26.1422, 1.6418) -> (-24.5959, 0.9818) centre (-21.5431, 10.2755) ccw projected
  arc A184 (-26.0928, 2.2972) -> (-26.1422, 1.6418) centre (0, 0) ccw projected
  arc A185 (-24.465, 2.7179) -> (-26.0928, 2.2972) centre (-22.8404, -6.9286) ccw projected
  arc A186 (-24.465, 2.7179) -> (-24.214, 2.9802) centre (-24.5154, 3.0173) ccw projected
  arc A187 (-24.2025, 3.0718) -> (-24.214, 2.9802) centre (0, 0) ccw projected
  arc A188 (-24.2025, 3.0718) -> (-24.3812, 3.3879) centre (-24.5038, 3.11) ccw projected
  arc A189 (-25.8554, 4.1963) -> (-24.3812, 3.3879) centre (-20.4322, 12.3376) ccw projected
  arc A190 (-25.742, 4.8437) -> (-25.8554, 4.1963) centre (0, 0) ccw projected
  arc A191 (-24.0808, 5.1028) -> (-25.742, 4.8437) centre (-23.4096, -4.6565) ccw projected
  arc A192 (-24.0808, 5.1028) -> (-23.8053, 5.3393) centre (-24.1016, 5.4057) ccw projected
  arc A193 (-23.7849, 5.4293) -> (-23.8053, 5.3393) centre (0, 0) ccw projected
  arc A194 (-23.7849, 5.4293) -> (-23.9317, 5.7614) centre (-24.081, 5.4969) ccw projected
  arc A195 (-25.3196, 6.7104) -> (-23.9317, 5.7614) centre (-19.1245, 14.2809) ccw projected
  arc A196 (-25.1433, 7.3435) -> (-25.3196, 6.7104) centre (0, 0) ccw projected
  arc A197 (-23.4646, 7.4385) -> (-25.1433, 7.3435) centre (-23.7533, -2.3395) ccw projected
  arc A198 (-23.4646, 7.4385) -> (-23.1673, 7.6469) centre (-23.4557, 7.7421) ccw projected
  arc A199 (-23.1382, 7.7345) -> (-23.1673, 7.6469) centre (0, 0) ccw projected
  arc A200 (-23.1382, 7.7345) -> (-23.2518, 8.0793) centre (-23.4262, 7.8307) ccw projected
  arc A201 (-24.54, 9.1598) -> (-23.2518, 8.0793) centre (-17.6326, 16.0867) ccw projected
  arc A202 (-24.3024, 9.7726) -> (-24.54, 9.1598) centre (0, 0) ccw projected
  arc A203 (-22.6226, 9.7026) -> (-24.3024, 9.7726) centre (-23.8682, 0) ccw projected
  arc A204 (-22.6226, 9.7026) -> (-22.3062, 9.8809) centre (-22.5839, 10.0039) ccw projected
  arc A205 (-22.2687, 9.9652) -> (-22.3062, 9.8809) centre (0, 0) ccw projected
  arc A206 (-22.2687, 9.9652) -> (-22.3479, 10.3195) centre (-22.5459, 10.0892) ccw projected
  arc A207 (-23.524, 11.5211) -> (-22.3479, 10.3195) centre (-15.9709, 17.7375) ccw projected
  arc A208 (-23.2275, 12.1076) -> (-23.524, 11.5211) centre (0, 0) ccw projected
  arc A209 (-21.5626, 11.8733) -> (-23.2275, 12.1076) centre (-23.7533, 2.3395) ccw projected
  arc A210 (-21.5626, 11.8733) -> (-21.2303, 12.0197) centre (-21.4946, 12.1693) ccw projected
  arc A211 (-21.1847, 12.0999) -> (-21.2303, 12.0197) centre (0, 0) ccw projected
  arc A212 (-21.1847, 12.0999) -> (-21.2288, 12.4603) centre (-21.4484, 12.2505) ccw projected
  arc A213 (-22.2814, 13.7713) -> (-21.2288, 12.4603) centre (-14.1555, 19.2175) ccw projected
  arc A214 (-21.9289, 14.326) -> (-22.2814, 13.7713) centre (0, 0) ccw projected
  arc A215 (-20.295, 13.9297) -> (-21.9289, 14.326) centre (-23.4096, 4.6565) ccw projected
  arc A216 (-20.295, 13.9297) -> (-19.95, 14.0427) centre (-20.1983, 14.2175) ccw projected
  arc A217 (-19.8967, 14.1181) -> (-19.95, 14.0427) centre (0, 0) ccw projected
  arc A218 (-19.8967, 14.1181) -> (-19.9053, 14.4811) centre (-20.1444, 14.2938) ccw projected
  arc A219 (-20.8243, 15.889) -> (-19.9053, 14.4811) centre (-12.2036, 20.5125) ccw projected
  arc A220 (-20.4191, 16.4065) -> (-20.8243, 15.889) centre (0, 0) ccw projected
  arc A221 (-18.8319, 15.8518) -> (-20.4191, 16.4065) centre (-22.8404, 6.9286) ccw projected
  arc A222 (-18.8319, 15.8518) -> (-18.4775, 15.9306) centre (-18.7075, 16.1289) ccw projected
  arc A223 (-18.4171, 16.0003) -> (-18.4775, 15.9306) centre (0, 0) ccw projected
  arc A224 (-18.4171, 16.0003) -> (-18.39, 16.3624) centre (-18.6463, 16.1995) ccw projected
  arc A225 (-19.1667, 17.8536) -> (-18.39, 16.3624) centre (-10.1343, 21.6099) ccw projected
  arc A226 (-18.7127, 18.3289) -> (-19.1667, 17.8536) centre (0, 0) ccw projected
  arc A227 (-17.1875, 17.6214) -> (-18.7127, 18.3289) centre (-22.0513, 9.134) ccw projected
  arc A228 (-17.1875, 17.6214) -> (-16.827, 17.6649) centre (-17.0365, 17.8848) ccw projected
  arc A229 (-16.7601, 17.7285) -> (-16.827, 17.6649) centre (0, 0) ccw projected
  arc A230 (-16.7601, 17.7285) -> (-16.6977, 18.0862) centre (-16.9687, 17.9492) ccw projected
  arc A231 (-17.3244, 19.6463) -> (-16.6977, 18.0862) centre (-7.9674, 22.4991) ccw projected
  arc A232 (-16.826, 20.0748) -> (-17.3244, 19.6463) centre (0, 0) ccw projected
  arc A233 (-15.3775, 19.2212) -> (-16.826, 20.0748) centre (-21.0499, 11.2514) ccw projected
  arc A234 (-15.3775, 19.2212) -> (-15.0145, 19.2292) centre (-15.2014, 19.4686) ccw projected
  arc A235 (-14.9417, 19.2859) -> (-15.0145, 19.2292) centre (0, 0) ccw projected
  arc A236 (-14.9417, 19.2859) -> (-14.8445, 19.6357) centre (-15.1277, 19.5259) ccw projected
  arc A237 (-15.3153, 21.2498) -> (-14.8445, 19.6357) centre (-5.7237, 23.1717) ccw projected
  arc A238 (-14.7773, 21.6274) -> (-15.3153, 21.2498) centre (0, 0) ccw projected
  arc A239 (-13.4195, 20.6359) -> (-14.7773, 21.6274) centre (-19.8457, 13.2605) ccw projected
  arc A240 (-13.4195, 20.6359) -> (-13.0574, 20.6083) centre (-13.22, 20.8648) ccw projected
  arc A241 (-12.9794, 20.6576) -> (-13.0574, 20.6083) centre (0, 0) ccw projected
  arc A242 (-12.9794, 20.6576) -> (-12.8484, 20.9962) centre (-13.141, 20.9147) ccw projected
  arc A243 (-13.1587, 22.6486) -> (-12.8484, 20.9962) centre (-3.4249, 23.6212) ccw projected
  arc A244 (-12.5863, 22.9716) -> (-13.1587, 22.6486) centre (0, 0) ccw projected
  arc A245 (-11.3322, 21.8518) -> (-12.5863, 22.9716) centre (-18.4504, 15.1418) ccw projected
  arc A246 (-11.3322, 21.8518) -> (-10.9746, 21.7889) centre (-11.1112, 22.0602) ccw projected
  arc A247 (-10.8921, 21.8303) -> (-10.9746, 21.7889) centre (0, 0) ccw projected
  arc A248 (-10.8921, 21.8303) -> (-10.7286, 22.1544) centre (-11.0277, 22.102) ccw projected
  arc A249 (-10.8754, 23.8294) -> (-10.7286, 22.1544) centre (-1.0931, 23.8431) ccw projected
  arc A250 (-10.2741, 24.0947) -> (-10.8754, 23.8294) centre (0, 0) ccw projected
  arc A251 (-9.1358, 22.8574) -> (-10.2741, 24.0947) centre (-16.8774, 16.8774) ccw projected
  arc A252 (-9.1358, 22.8574) -> (-8.7861, 22.7597) centre (-8.8954, 23.043) ccw projected
  arc A253 (-8.6999, 22.7928) -> (-8.7861, 22.7597) centre (0, 0) ccw projected
  arc A254 (-8.6999, 22.7928) -> (-8.5054, 23.0994) centre (-8.8082, 23.0765) ccw projected
  arc A255 (-8.4873, 24.7806) -> (-8.5054, 23.0994) centre (1.2492, 23.8355) ccw projected
  arc A256 (-7.863, 24.9857) -> (-8.4873, 24.7806) centre (0, 0) ccw projected
  arc A257 (-6.8514, 23.6428) -> (-7.863, 24.9857) centre (-15.1418, 18.4504) ccw projected
  arc A258 (-6.8514, 23.6428) -> (-6.5129, 23.5113) centre (-6.594, 23.804) ccw projected
  arc A259 (-6.4239, 23.5358) -> (-6.5129, 23.5113) centre (0, 0) ccw projected
  arc A260 (-6.4239, 23.5358) -> (-6.2003, 23.8218) centre (-6.5039, 23.8287) ccw projected
  arc A261 (-6.0176, 25.4932) -> (-6.2003, 23.8218) centre (3.5794, 23.5983) ccw projected
  arc A262 (-5.3761, 25.6361) -> (-6.0176, 25.4932) centre (0, 0) ccw projected
  arc A263 (-4.501, 24.2005) -> (-5.3761, 25.6361) centre (-13.2605, 19.8457) ccw projected
  arc A264 (-4.501, 24.2005) -> (-4.177, 24.0365) centre (-4.229, 24.3357) ccw projected
  arc A265 (-4.0861, 24.0521) -> (-4.177, 24.0365) centre (0, 0) ccw projected
  arc A266 (-4.0861, 24.0521) -> (-3.8355, 24.3148) centre (-4.137, 24.3515) ccw projected
  arc A267 (-3.4898, 25.9602) -> (-3.8355, 24.3148) centre (5.8752, 23.1338) ccw projected
  arc A268 (-2.8374, 26.0396) -> (-3.4898, 25.9602) centre (0, 0) ccw projected
  arc A269 (-2.1072, 24.5251) -> (-2.8374, 26.0396) centre (-11.2514, 21.0499) ccw projected
  arc A270 (-2.1072, 24.5251) -> (-1.8009, 24.3301) centre (-1.8234, 24.633) ccw projected
  arc A271 (-1.7089, 24.3368) -> (-1.8009, 24.3301) centre (0, 0) ccw projected
  arc A272 (-1.7089, 24.3368) -> (-1.4337, 24.5737) centre (-1.7302, 24.6397) ccw projected
  arc A273 (-0.9285, 26.1773) -> (-1.4337, 24.5737) centre (8.1145, 22.4465) ccw projected
  arc A274 (-0.2714, 26.1923) -> (-0.9285, 26.1773) centre (0, 0) ccw projected
  arc A275 (0.3068, 24.6136) -> (-0.2714, 26.1923) centre (-9.134, 22.0513) ccw projected
  arc A276 (0.3068, 24.6136) -> (0.5925, 24.3895) centre (0.5999, 24.6931) ccw projected
  arc A277 (0.6848, 24.3871) -> (0.5925, 24.3895) centre (0, 0) ccw projected
  arc A278 (0.6848, 24.3871) -> (0.9818, 24.5959) centre (0.6933, 24.6907) ccw projected
  arc A279 (1.6418, 26.1422) -> (0.9818, 24.5959) centre (10.2755, 21.5431) ccw projected
  arc A280 (2.2972, 26.0928) -> (1.6418, 26.1422) centre (0, 0) ccw projected
  arc A281 (2.7179, 24.465) -> (2.2972, 26.0928) centre (-6.9286, 22.8404) ccw projected
  arc A282 (2.7179, 24.465) -> (2.9802, 24.214) centre (3.0173, 24.5154) ccw projected
  arc A283 (3.0718, 24.2025) -> (2.9802, 24.214) centre (0, 0) ccw projected
  arc A284 (3.0718, 24.2025) -> (3.3879, 24.3812) centre (3.11, 24.5038) ccw projected
  arc A285 (4.1963, 25.8554) -> (3.3879, 24.3812) centre (12.3376, 20.4322) ccw projected
  arc A286 (4.8437, 25.742) -> (4.1963, 25.8554) centre (0, 0) ccw projected
  arc A287 (5.1028, 24.0808) -> (4.8437, 25.742) centre (-4.6565, 23.4096) ccw projected
  arc A288 (5.1028, 24.0808) -> (5.3393, 23.8053) centre (5.4057, 24.1016) ccw projected
  arc A289 (5.4293, 23.7849) -> (5.3393, 23.8053) centre (0, 0) ccw projected
  arc A290 (5.4293, 23.7849) -> (5.7614, 23.9317) centre (5.4969, 24.081) ccw projected
  arc A291 (6.7104, 25.3196) -> (5.7614, 23.9317) centre (14.2809, 19.1245) ccw projected
  arc A292 (7.3435, 25.1433) -> (6.7104, 25.3196) centre (0, 0) ccw projected
  arc A293 (7.4385, 23.4646) -> (7.3435, 25.1433) centre (-2.3395, 23.7533) ccw projected
  arc A294 (7.4385, 23.4646) -> (7.6469, 23.1673) centre (7.7421, 23.4557) ccw projected
  arc A295 (7.7345, 23.1382) -> (7.6469, 23.1673) centre (0, 0) ccw projected
  arc A296 (7.7345, 23.1382) -> (8.0793, 23.2518) centre (7.8307, 23.4262) ccw projected
  arc A297 (9.1598, 24.54) -> (8.0793, 23.2518) centre (16.0867, 17.6326) ccw projected
  arc A298 (9.7726, 24.3024) -> (9.1598, 24.54) centre (0, 0) ccw projected
  arc A299 (9.7026, 22.6226) -> (9.7726, 24.3024) centre (0, 23.8682) ccw projected
  arc A300 (9.7026, 22.6226) -> (9.8809, 22.3062) centre (10.0039, 22.5839) ccw projected
  arc A301 (9.9652, 22.2687) -> (9.8809, 22.3062) centre (0, 0) ccw projected
  arc A302 (9.9652, 22.2687) -> (10.3195, 22.3479) centre (10.0892, 22.5459) ccw projected
  arc A303 (11.5211, 23.524) -> (10.3195, 22.3479) centre (17.7375, 15.9709) ccw projected
  arc A304 (12.1076, 23.2275) -> (11.5211, 23.524) centre (0, 0) ccw projected
  arc A305 (11.8733, 21.5626) -> (12.1076, 23.2275) centre (2.3395, 23.7533) ccw projected
  arc A306 (11.8733, 21.5626) -> (12.0197, 21.2303) centre (12.1693, 21.4946) ccw projected
  arc A307 (12.0999, 21.1847) -> (12.0197, 21.2303) centre (0, 0) ccw projected
  arc A308 (12.0999, 21.1847) -> (12.4603, 21.2288) centre (12.2505, 21.4484) ccw projected
  arc A309 (13.7713, 22.2814) -> (12.4603, 21.2288) centre (19.2175, 14.1555) ccw projected
  arc A310 (14.326, 21.9289) -> (13.7713, 22.2814) centre (0, 0) ccw projected
  arc A311 (13.9297, 20.295) -> (14.326, 21.9289) centre (4.6565, 23.4096) ccw projected
  arc A312 (13.9297, 20.295) -> (14.0427, 19.95) centre (14.2175, 20.1983) ccw projected
  arc A313 (14.1181, 19.8967) -> (14.0427, 19.95) centre (0, 0) ccw projected
  arc A314 (14.1181, 19.8967) -> (14.4811, 19.9053) centre (14.2938, 20.1444) ccw projected
  arc A315 (15.889, 20.8243) -> (14.4811, 19.9053) centre (20.5125, 12.2036) ccw projected
  arc A316 (16.4065, 20.4191) -> (15.889, 20.8243) centre (0, 0) ccw projected
  arc A317 (15.8518, 18.8319) -> (16.4065, 20.4191) centre (6.9286, 22.8404) ccw projected
  arc A318 (15.8518, 18.8319) -> (15.9306, 18.4775) centre (16.1289, 18.7075) ccw projected
  arc A319 (16.0003, 18.4171) -> (15.9306, 18.4775) centre (0, 0) ccw projected
  arc A320 (16.0003, 18.4171) -> (16.3624, 18.39) centre (16.1995, 18.6463) ccw projected
  arc A321 (17.8536, 19.1667) -> (16.3624, 18.39) centre (21.6099, 10.1343) ccw projected
  arc A322 (18.3289, 18.7127) -> (17.8536, 19.1667) centre (0, 0) ccw projected
  arc A323 (17.6214, 17.1875) -> (18.3289, 18.7127) centre (9.134, 22.0513) ccw projected
  arc A324 (17.6214, 17.1875) -> (17.6649, 16.827) centre (17.8848, 17.0365) ccw projected
  arc A325 (17.7285, 16.7601) -> (17.6649, 16.827) centre (0, 0) ccw projected
  arc A326 (17.7285, 16.7601) -> (18.0862, 16.6977) centre (17.9492, 16.9687) ccw projected
  arc A327 (19.6463, 17.3244) -> (18.0862, 16.6977) centre (22.4991, 7.9674) ccw projected
  arc A328 (20.0748, 16.826) -> (19.6463, 17.3244) centre (0, 0) ccw projected
  arc A329 (19.2212, 15.3775) -> (20.0748, 16.826) centre (11.2514, 21.0499) ccw projected
  arc A330 (19.2212, 15.3775) -> (19.2292, 15.0145) centre (19.4686, 15.2014) ccw projected
  arc A331 (19.2859, 14.9417) -> (19.2292, 15.0145) centre (0, 0) ccw projected
  arc A332 (19.2859, 14.9417) -> (19.6357, 14.8445) centre (19.5259, 15.1277) ccw projected
  arc A333 (21.2498, 15.3153) -> (19.6357, 14.8445) centre (23.1717, 5.7237) ccw projected
  arc A334 (21.6274, 14.7773) -> (21.2498, 15.3153) centre (0, 0) ccw projected
  arc A335 (20.6359, 13.4195) -> (21.6274, 14.7773) centre (13.2605, 19.8457) ccw projected
  arc A336 (20.6359, 13.4195) -> (20.6083, 13.0574) centre (20.8648, 13.22) ccw projected
  arc A337 (20.6576, 12.9794) -> (20.6083, 13.0574) centre (0, 0) ccw projected
  arc A338 (20.6576, 12.9794) -> (20.9962, 12.8484) centre (20.9147, 13.141) ccw projected
  arc A339 (22.6486, 13.1587) -> (20.9962, 12.8484) centre (23.6212, 3.4249) ccw projected
  arc A340 (22.9716, 12.5863) -> (22.6486, 13.1587) centre (0, 0) ccw projected
  arc A341 (21.8518, 11.3322) -> (22.9716, 12.5863) centre (15.1418, 18.4504) ccw projected
  arc A342 (21.8518, 11.3322) -> (21.7889, 10.9746) centre (22.0602, 11.1112) ccw projected
  arc A343 (21.8303, 10.8921) -> (21.7889, 10.9746) centre (0, 0) ccw projected
  arc A344 (21.8303, 10.8921) -> (22.1544, 10.7286) centre (22.102, 11.0277) ccw projected
  arc A345 (23.8294, 10.8754) -> (22.1544, 10.7286) centre (23.8431, 1.0931) ccw projected
  arc A346 (24.0947, 10.2741) -> (23.8294, 10.8754) centre (0, 0) ccw projected
  arc A347 (22.8574, 9.1358) -> (24.0947, 10.2741) centre (16.8774, 16.8774) ccw projected
  arc A348 (22.8574, 9.1358) -> (22.7597, 8.7861) centre (23.043, 8.8954) ccw projected
  arc A349 (22.7928, 8.6999) -> (22.7597, 8.7861) centre (0, 0) ccw projected
  arc A350 (22.7928, 8.6999) -> (23.0994, 8.5054) centre (23.0765, 8.8082) ccw projected
  arc A351 (24.7806, 8.4873) -> (23.0994, 8.5054) centre (23.8355, -1.2492) ccw projected
  arc A352 (24.9857, 7.863) -> (24.7806, 8.4873) centre (0, 0) ccw projected
  arc A353 (23.6428, 6.8514) -> (24.9857, 7.863) centre (18.4504, 15.1418) ccw projected
  arc A354 (23.6428, 6.8514) -> (23.5113, 6.5129) centre (23.804, 6.594) ccw projected
  arc A355 (23.5358, 6.4239) -> (23.5113, 6.5129) centre (0, 0) ccw projected
  arc A356 (23.5358, 6.4239) -> (23.8218, 6.2003) centre (23.8287, 6.5039) ccw projected
  arc A357 (25.4932, 6.0176) -> (23.8218, 6.2003) centre (23.5983, -3.5794) ccw projected
  arc A358 (25.6361, 5.3761) -> (25.4932, 6.0176) centre (0, 0) ccw projected
  arc A359 (24.2005, 4.501) -> (25.6361, 5.3761) centre (19.8457, 13.2605) ccw projected
  arc A360 (24.2005, 4.501) -> (24.0365, 4.177) centre (24.3357, 4.229) ccw projected
  arc A361 (24.0521, 4.0861) -> (24.0365, 4.177) centre (0, 0) ccw projected
  arc A362 (24.0521, 4.0861) -> (24.3148, 3.8355) centre (24.3515, 4.137) ccw projected
  arc A363 (25.9602, 3.4898) -> (24.3148, 3.8355) centre (23.1338, -5.8752) ccw projected
  arc A364 (26.0396, 2.8374) -> (25.9602, 3.4898) centre (0, 0) ccw projected
  arc A365 (24.5251, 2.1072) -> (26.0396, 2.8374) centre (21.0499, 11.2514) ccw projected
  arc A366 (24.5251, 2.1072) -> (24.3301, 1.8009) centre (24.633, 1.8234) ccw projected
  arc A367 (24.3368, 1.7089) -> (24.3301, 1.8009) centre (0, 0) ccw projected
  arc A368 (24.3368, 1.7089) -> (24.5737, 1.4337) centre (24.6397, 1.7302) ccw projected
  arc A369 (26.1773, 0.9285) -> (24.5737, 1.4337) centre (22.4465, -8.1145) ccw projected
  arc A370 (26.1923, 0.2714) -> (26.1773, 0.9285) centre (0, 0) ccw projected
  arc A371 (24.6136, -0.3068) -> (26.1923, 0.2714) centre (22.0513, 9.134) ccw projected
  arc A372 (24.6136, -0.3068) -> (24.3895, -0.5925) centre (24.6931, -0.5999) ccw projected
  arc A373 (24.3871, -0.6848) -> (24.3895, -0.5925) centre (0, 0) ccw projected
  arc A374 (24.3871, -0.6848) -> (24.5959, -0.9818) centre (24.6907, -0.6933) ccw projected
  arc A375 (26.1422, -1.6418) -> (24.5959, -0.9818) centre (21.5431, -10.2755) ccw projected
  arc A376 (26.0928, -2.2972) -> (26.1422, -1.6418) centre (0, 0) ccw projected
  arc A377 (24.465, -2.7179) -> (26.0928, -2.2972) centre (22.8404, 6.9286) ccw projected
  arc A378 (24.465, -2.7179) -> (24.214, -2.9802) centre (24.5154, -3.0173) ccw projected
  arc A379 (24.2025, -3.0718) -> (24.214, -2.9802) centre (0, 0) ccw projected
  arc A380 (24.2025, -3.0718) -> (24.3812, -3.3879) centre (24.5038, -3.11) ccw projected
  arc A381 (25.8554, -4.1963) -> (24.3812, -3.3879) centre (20.4322, -12.3376) ccw projected
  arc A382 (25.742, -4.8437) -> (25.8554, -4.1963) centre (0, 0) ccw projected
  arc A383 (24.0808, -5.1028) -> (25.742, -4.8437) centre (23.4096, 4.6565) ccw projected
  circle A384 centre (0, 0) radius 29.475 projected
  point P0 (0, 0)
extrude "Extrusion7" add sketch "Sketch7" along normal blind 5.08
sketch "Sketch8" plane through (0, 0, 25.781) normal (0, 0, 1) x (1, 0, 0)
  circle A0 centre (0, 0) radius 5.715
  dimension "d18" = 11.43
  constraints: 1 centre point, 1 coincident
  measures "d18" diameter of A0
extrude "Extrusion8" cut sketch "Sketch8" against normal blind 5.08
sketch "Sketch9" plane through (0, 0, 37.211) normal (0, 0, 1) x (1, 0, 0)
  circle A0 centre (0, 33.02) radius 1.778
  circle A1 centre (0, 0) radius 29.475 projected
  circle A2 centre (0, 33.02) radius 5.588
  line L0 (0, -43.3048) -> (0, 53.5037) projected
  circle A3 centre (0, 33.02) radius 1.778
  circle A4 centre (0, 33.02) radius 5.588
  circle A5 centre (0, 33.02) radius 1.778
  circle A6 centre (0, 33.02) radius 5.588
  circle A7 centre (0, 33.02) radius 1.778
  circle A8 centre (0, 33.02) radius 5.588
  circle A9 centre (0, 33.02) radius 1.778
  circle A10 centre (0, 33.02) radius 5.588
  circle A11 centre (0, 33.02) radius 1.778
  circle A12 centre (0, 33.02) radius 5.588
  circle A13 centre (0, 33.02) radius 1.778
  circle A14 centre (0, 33.02) radius 5.588
  circle A15 centre (0, 33.02) radius 1.778
  circle A16 centre (0, 33.02) radius 5.588
  circle A17 centre (0, 33.02) radius 5.588
  circle A18 centre (0, 33.02) radius 1.778
  circle A19 centre (0, 33.02) radius 5.588
  circle A20 centre (0, 33.02) radius 1.778
  circle A21 centre (0, 33.02) radius 5.588
  circle A22 centre (0, 33.02) radius 1.778
  line L1 (0, 0) -> (5.715, 0)
  circle A23 centre (0, 0) radius 5.715 projected
  line L2 (0, 0) -> (7.2493, -7.2493) construction
  circle A24 centre (0, -33.02) radius 1.778
  circle A25 centre (0, -33.02) radius 5.588
  circle A26 centre (-33.02, 0) radius 1.778
  circle A27 centre (-33.02, 0) radius 5.588
  circle A28 centre (33.02, 0) radius 1.778
  circle A29 centre (33.02, 0) radius 5.588
  dimension "d21" = 3.81
  dimension "d22" = 3.556
  dimension "d23" = 33.02
  dimension "d26" = 0
  dimension "d30" = 0
  dimension "d34" = 0
  dimension "d36" = 45
  constraints: 28 centre point, 14 coincident, 6 symmetric about line, 4 end point, 1 horizontal, 1 horizontal alignment, 1 point on line, 50 other
  measures "d21" radial gap between concentric circles of A2 A0
  measures "d22" diameter of A0
  measures "d23" distance of L1.start A0.centre
  measures "d36" angle of L0 L2
extrude "Extrusion9" add sketch "Sketch9" against normal up to surface (12.7 mm away) contours A0 L0 A2 A1 | A0 L0 A1 A2 | L0 A2 A1 | A1 A2 L0 | A27 A1 | A1 A27 | A29 A1 | A1 A29 | A25 L0 A1 | A1 L0 A24 A25 | A25 L0 A24 A1 | A1 L0 A25